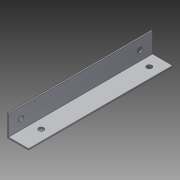
# Autodesk Inventor part: Hopper Bracing P2
Saved by Autodesk Inventor 2014 SP1 (Build 180222100, 222)
## iProperties
Created: 2013-12-16
Part Number: Hopper Bracing P2
Material: Aluminum 6061
Document SubType Name: Modeling
Designer: Moses
Mass: 7.09017 g
Surface Area: 68.5076 cm^2
Volume: 2.6163 cm^3
Density: 2.71 g/cm^3
Appearance: Aluminum - Flat
Author: Moses
Autodesk Inventor part; units mm, degrees
ref_plane "YZ Plane" through (0, 0, 0) normal (1, 0, 0) x (0, 1, 0)
ref_plane "XZ Plane" through (0, 0, 0) normal (0, 1, 0) x (-1, 0, 0)
ref_plane "XY Plane" through (0, 0, 0) normal (0, 0, 1) x (1, 0, 0)
sketch "Sketch1" plane through (0, 0, 0) normal (0, 0, 1) x (1, 0, 0)
  line L0 (0, 0) -> (0, 15.875)
  line L1 (0, 15.875) -> (0.7937, 15.875)
  line L2 (0.7937, 15.875) -> (0.7938, 0.7937)
  line L3 (0.7938, 0.7937) -> (15.875, 0.7937)
  line L4 (15.875, 0.7937) -> (15.875, 0)
  line L5 (15.875, 0) -> (0, 0)
  dimension "d0" = 15.875
  dimension "d1" = 0.7937
  constraints: 12 end point, 3 horizontal, 3 vertical, 2 perpendicular
  measures "d0" distance of L0.start L0.end
  measures "d1" distance of L0.end L1.end
extrude "Extrusion1" add sketch "Sketch1" along normal blind 107.95
sketch "Sketch2" plane through (0, 0, 0) normal (0, -1, 0) x (1, 0, 0)
  line L0 (15.875, 0) -> (0, 0) projected
  line L1 (0, 107.95) -> (15.875, 107.95) projected
  line L2 (7.9375, 107.95) -> (7.9375, 0) construction
  circle A0 centre (7.9375, 90.4875) radius 1.905
  circle A1 centre (7.9375, 9.525) radius 1.905
  line L3 (257.175, 98.425) -> (-9.525, 98.425) construction
  line L4 (-15.875, 82.55) -> (187.325, 82.55) construction
  dimension "d4" = 3.81
  dimension "d6" = 17.4625
  dimension "d7" = 9.525
  dimension "d16" = 15.875
  dimension "d17" = 9.525
  constraints: 2 centre point, 2 end point, 2 midpoint, 2 point on line, 1 equal radius
  measures "d4" diameter of A0
  measures "d6" distance from line of L1 A0.centre
  measures "d7" distance of L2.end A1.centre
  measures "d16" distance between parallel lines of L4 L3
  measures "d17" distance between parallel lines of L1 L3
extrude "Extrusion2" cut sketch "Sketch2" against normal through all
sketch "Sketch3" plane through (0, 0, 0) normal (-1, 0, 0) x (0, 0, 1)
  line L0 (0, 0) -> (0, 15.875) projected
  line L1 (107.95, 15.875) -> (107.95, 0) projected
  line L2 (0, 7.9375) -> (107.95, 7.9375) construction
  circle A0 centre (9.525, 7.9375) radius 1.905
  circle A1 centre (98.425, 7.9375) radius 1.905
  dimension "d11" = 3.81
  dimension "d12" = 9.525
  dimension "d13" = 9.525
  constraints: 2 centre point, 2 end point, 2 midpoint, 2 point on line, 1 equal radius
  measures "d11" diameter of A1
  measures "d12" distance from line of L1 A1.centre
  measures "d13" distance from line of L0 A0.centre
extrude "Extrusion3" cut sketch "Sketch3" against normal through all
equation "\"d6\" = d17 + 0.5 * d16"
body "Solid1"
